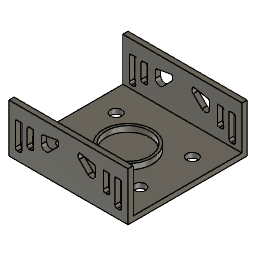
Gantry Car (Autodesk Fusion 360 design; units mm, degrees)
part number: 2026-04-23-20-09-53-630
Autodesk Fusion 360 part; units mm, degrees
sketch "Sketch1" plane through (0, 0, 0) normal (0, 0, 1) x (1, 0, 0)
  line L0 (-4.2629, 5.2747) -> (50.7371, 5.2747)
  line L1 (50.7371, 5.2747) -> (50.7371, -49.7253)
  line L2 (50.7371, -49.7253) -> (-4.2629, -49.7253)
  line L3 (-4.2629, -49.7253) -> (-4.2629, 5.2747)
  line L4 (-4.2629, 5.2747) -> (50.7371, 5.2747)
  line L5 (50.7371, 5.2747) -> (50.7371, 2.8747)
  line L6 (50.7371, 2.8747) -> (-4.2629, 2.8747)
  line L7 (-4.2629, 2.8747) -> (-4.2629, 5.2747)
  line L8 (-4.2629, -49.7253) -> (50.7371, -49.7253)
  line L9 (50.7371, -49.7253) -> (50.7371, -47.3253)
  line L10 (50.7371, -47.3253) -> (-4.2629, -47.3253)
  line L11 (-4.2629, -47.3253) -> (-4.2629, -49.7253)
  circle A0 centre (23.2371, -22.2253) radius 10.1
  circle A1 centre (23.2371, -22.2253) radius 11.3
  dimension "d1" = 55
  dimension "d2" = 55
  dimension "d3" = 2.4
  dimension "d4" = 2.4
  dimension "d9" = 20.2
  dimension "d10" = 27.5
  dimension "d11" = 27.5
  dimension "d12" = 22.6
  constraint horizontal L0
  constraint vertical L1
  constraint horizontal L2
  constraint vertical L3
  constraint horizontal L4
  constraint vertical L5
  constraint horizontal L6
  constraint vertical L7
  constraint horizontal L8
  constraint vertical L9
  constraint horizontal L10
  constraint vertical L11
  constraint coincident L1 L9.end
  constraint concentric A0 A1
  measures "d1" distance of L0.start L2.end
  measures "d2" distance of L0.start L0.end
  measures "d3" distance of L0.start L6.end
  measures "d4" distance of L1.end L9.end
  measures "d9" diameter of A0
  measures "d10" distance of L8 A0.centre
  measures "d11" distance of L1 A0.centre
  measures "d12" diameter of A1
extrude "Extrude4" add sketch "Sketch1" along normal blind 32.4 contours L0 L1 L3 L4 L5 L6 L7 | L1 L2 L3 L8 L9 L10 L11 makes body 1 at (14.0704, 5.2747, 10.8) makes body 2 at (32.4037, -47.3253, 10.8)
extrude "Extrude5" add sketch "Sketch1" along normal blind 2.4 separate body contours A0 makes body 3
extrude "Extrude6" add sketch "Sketch1" along normal blind 2.4 contours L1 L3 L6 L10 bodies 1 2
extrude "Extrude7" add sketch "Sketch1" along normal blind 5 contours A1 bodies 1 3
sketch "Sketch2" plane through (0, 5.2747, 0) normal (0, 1, 0) x (-1, 0, 0)
  line L0 (-50.7371, 0) -> (4.2629, 0)
  line L1 (4.2629, 0) -> (4.2629, 32.4)
  line L2 (4.2629, 32.4) -> (-50.7371, 32.4)
  line L3 (-50.7371, 32.4) -> (-50.7371, 0)
  line L4 (-44.7371, 16.2) -> (-47.7371, 16.2)
  line L5 (-39.3371, 16.2) -> (-41.5871, 16.2)
  line L6 (-47.7371, 5) -> (-44.7371, 5)
  arc A0 (-42.3371, 8.4246) -> (-41.3371, 7.4246) centre (-41.3371, 8.4246) ccw
  arc A1 (-35.6811, 12.233) -> (-32.2659, 10.8198) centre (-33.6811, 12.233) ccw
  line L7 (-41.3371, 7.4246) -> (-40.3371, 7.4246)
  arc A2 (-47.7371, 5) -> (-46.7371, 4) centre (-46.7371, 5) ccw
  arc A3 (-45.7371, 4) -> (-44.7371, 5) centre (-45.7371, 5) ccw
  arc A4 (-40.3371, 7.4246) -> (-39.3371, 8.4246) centre (-40.3371, 8.4246) ccw
  line L8 (-46.7371, 4) -> (-45.7371, 4)
  line L9 (-44.7371, 5) -> (-44.7371, 16.2)
  line L10 (-42.3371, 15.45) -> (-42.3371, 8.4246)
  line L11 (-32.2659, 10.8198) -> (-28.2346, 14.8565)
  line L12 (-47.7371, 15.45) -> (-47.7371, 5)
  line L13 (-44.7371, 16.2) -> (-46.9871, 16.2)
  line L14 (-35.6811, 15.3643) -> (-35.6811, 12.233)
  line L15 (-39.3371, 8.4246) -> (-39.3371, 16.2)
  arc A5 (-28.2346, 14.8565) -> (-28.2346, 17.5435) centre (-29.5799, 16.2) ccw
  line L16 (1.2629, 15.45) -> (1.2629, 5)
  arc A6 (-7.1371, 8.4246) -> (-6.1371, 7.4246) centre (-6.1371, 8.4246) ccw
  line L17 (-1.7371, 5) -> (-1.7371, 16.2)
  arc A7 (-18.2396, 17.5435) -> (-18.2396, 14.8565) centre (-16.8943, 16.2) ccw
  line L18 (-7.1371, 8.4246) -> (-7.1371, 16.2)
  line L19 (-14.2082, 10.8198) -> (-18.2396, 14.8565)
  line L20 (-7.1371, 16.2) -> (-5.1371, 16.2)
  line L21 (-10.7931, 15.5732) -> (-10.7931, 12.233)
  line L22 (-5.1371, 7.4246) -> (-6.1371, 7.4246)
  arc A8 (0.2629, 4) -> (1.2629, 5) centre (0.2629, 5) ccw
  arc A9 (-1.7371, 5) -> (-0.7371, 4) centre (-0.7371, 5) ccw
  arc A10 (-5.1371, 7.4246) -> (-4.1371, 8.4246) centre (-5.1371, 8.4246) ccw
  line L23 (-4.1371, 15.2) -> (-4.1371, 8.4246)
  line L24 (0.2629, 4) -> (-0.7371, 4)
  line L25 (-1.7371, 16.2) -> (0.5129, 16.2)
  arc A11 (-14.2082, 10.8198) -> (-10.7931, 12.233) centre (-12.7931, 12.233) ccw
  line L26 (1.2629, 5) -> (-1.7371, 5)
  line L27 (-34.8586, 16.3484) -> (-28.2346, 17.5435)
  line L28 (-18.2396, 17.5435) -> (-11.4099, 16.3113)
  arc A12 (-34.8586, 16.3484) -> (-35.6811, 15.3643) centre (-34.6811, 15.3643) ccw
  arc A13 (-4.1371, 15.2) -> (-5.1371, 16.2) centre (-5.1371, 15.2) ccw
  arc A14 (1.2629, 15.45) -> (0.5129, 16.2) centre (0.5129, 15.45) ccw
  arc A15 (-10.7931, 15.5732) -> (-11.4099, 16.3113) centre (-11.5431, 15.5732) ccw
  arc A16 (-46.9871, 16.2) -> (-47.7371, 15.45) centre (-46.9871, 15.45) ccw
  arc A17 (-41.5871, 16.2) -> (-42.3371, 15.45) centre (-41.5871, 15.45) ccw
  point P0 (-50.7371, 0)
  point P1 (4.2629, 32.4)
  dimension "d40" = 1.9013
  dimension "d61" = 1
  dimension "d62" = 1
  dimension "d63" = 0.75
  constraint horizontal L4
  constraint horizontal L5
  constraint tangent L11 A5
  constraint tangent L14 A12
  constraint tangent L27 A12
  constraint tangent L20 A13
  constraint tangent L23 A13
  constraint tangent L16 A14
  constraint tangent L25 A14
  constraint tangent L21 A15
  constraint tangent L28 A15
  constraint equal A14 A15
  constraint tangent L12 A16
  constraint tangent L13 A16
  constraint equal A14 A16
  constraint tangent L10 A17
  constraint tangent L5 A17
  constraint equal A14 A17
  measures "d40" radius of A5
  measures "d61" radius of A12
  measures "d62" radius of A13
  measures "d63" radius of A14
extrude "Extrude8" cut sketch "Sketch2" against normal blind 56 contours L4 L6 L9 L12 L13 A16 | L6 A2 A3 L8 | L5 A0 L7 A4 L10 L15 A17 | A1 L11 L14 A5 L27 A12 | L16 L17 L25 L26 A14 | A8 A9 L24 L26 | A6 L18 L20 L22 A10 L23 A13 | A7 L19 L21 A11 L28 A15 bodies 1
sketch "Sketch3" plane through (0, 0, 2.4) normal (0, 0, 1) x (-1, 0, 0)
  circle A0 centre (-23.2371, 22.2253) radius 11.3
  line L0 (-50.7371, -2.8747) -> (4.2629, -2.8747)
  line L1 (4.2629, -2.8747) -> (4.2629, 47.3253)
  line L2 (4.2629, 47.3253) -> (-50.7371, 47.3253)
  line L3 (-50.7371, 47.3253) -> (-50.7371, -2.8747)
  circle A1 centre (-5.6371, 10.1253) radius 2.6
  line L4 (-44.8671, 22.2253) -> (-44.3164, 22.2253)
  circle A2 centre (-5.6371, 34.3253) radius 2.6
  circle A3 centre (-40.8371, 34.3253) radius 2.6
  circle A4 centre (-40.8371, 10.1253) radius 2.6
  dimension "d43" = 5.2
  dimension "d47" = 13
  dimension "d48" = 9.9
  dimension "d49" = 9.9
  dimension "d50" = 9.9
  dimension "d51" = 9.9
  dimension "d54" = 13
  dimension "d55" = 13
  dimension "d56" = 13
  constraint horizontal L4
  measures "d43" diameter of A1
  measures "d47" distance of L0 A1.centre
  measures "d48" distance of L1 A1.centre
  measures "d49" distance of L1 A2.centre
  measures "d50" distance of L3 A3.centre
  measures "d51" distance of L3 A4.centre
  measures "d54" distance of L2 A2.centre
  measures "d55" distance of L2 A3.centre
  measures "d56" distance of L0 A4.centre
extrude "Extrude9" cut sketch "Sketch3" against normal blind 2.5 contours A1 | A2 | A3 | A4 bodies 1
extrude "Extrude10" cut 2 faces at (14.0704, -48.9253, 32.4) (14.0704, 4.4747, 32.4) along direction (0, 0, -1) blind 10 on bodies 1 bodies 1
delete_face "DeleteFace1" 2 faces at (0.9871, -48.1253, 16.2) (0.9871, 4.4747, 16.2) on bodies 1
